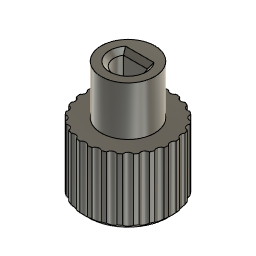
volume-knob (Autodesk Fusion 360 design; units mm, degrees)
Autodesk Fusion 360 part; units mm, degrees
note: some values were not read from the file. Set by a fixed rule: which sketch regions a step uses.
sketch "Skizze1" plane through (0, 0, 0) normal (0, 0, 1) x (1, 0, 0)
  circle A0 centre (0, 0) radius 10
  circle A1 centre (0, 10.5) radius 1
  circle A2 centre (-2.7176, 10.1422) radius 1
  circle A3 centre (-5.25, 9.0933) radius 1
  circle A4 centre (-7.4246, 7.4246) radius 1
  circle A5 centre (-9.0933, 5.25) radius 1
  circle A6 centre (-10.1422, 2.7176) radius 1
  circle A7 centre (-10.5, 0) radius 1
  circle A8 centre (-10.1422, -2.7176) radius 1
  circle A9 centre (-9.0933, -5.25) radius 1
  circle A10 centre (-7.4246, -7.4246) radius 1
  circle A11 centre (-5.25, -9.0933) radius 1
  circle A12 centre (-2.7176, -10.1422) radius 1
  circle A13 centre (0, -10.5) radius 1
  circle A14 centre (2.7176, -10.1422) radius 1
  circle A15 centre (5.25, -9.0933) radius 1
  circle A16 centre (7.4246, -7.4246) radius 1
  circle A17 centre (9.0933, -5.25) radius 1
  circle A18 centre (10.1422, -2.7176) radius 1
  circle A19 centre (10.5, 0) radius 1
  circle A20 centre (10.1422, 2.7176) radius 1
  circle A21 centre (9.0933, 5.25) radius 1
  circle A22 centre (7.4246, 7.4246) radius 1
  circle A23 centre (5.25, 9.0933) radius 1
  circle A24 centre (2.7176, 10.1422) radius 1
  dimension "d1" = 20
  dimension "d2" = 2
  dimension "d4" = 360
  dimension "d7" = 10.5
  constraint coincident A0.centre origin
  measures "d1" diameter of A0
  measures "d2" diameter of A1
  measures "d7" distance of A0.centre A1.centre
extrude "Extrusion1" add sketch "Skizze1" along normal blind 15 contours A0 A1 A2 A3 A4 A5 A6 A7 A8 A9 A10 A11 A12 A13 A14 A15 A16 A17 A18 A19 A20 A21 A22 A23 A24
sketch "Skizze3" plane through (0, 0, 0) normal (0, 1, 0) x (1, 0, 0)
  line L0 (10.9643, -2.0711) -> (7.9643, 0.9289)
  line L1 (7.9643, 0.9289) -> (10.9643, 0.9289)
  line L2 (10.9643, 0.9289) -> (10.9643, -2.0711)
  point P0 (9.9643, 0)
  dimension "d10" = 3
  dimension "d11" = 3
  dimension "d12" = 1
  constraint horizontal L1
  constraint perpendicular L1 L2
  measures "d10" distance of L0.end L1.end
  measures "d11" distance of L0.start L1.end
  measures "d12" distance of L2 P0
revolve "Drehen1" cut sketch "Skizze3" angle 360 about axis through (0, 0, 1.75) along (0, 0, 1)
sketch "Skizze4" plane through (0, 0, 15) normal (0, 0, 1) x (-1, 0, 0)
  arc A0 (-6.4487, -7.6429) -> (-5.7134, -8.2071) centre (0, 0) ccw
  arc A1 (-4.2509, -9.0515) -> (-5.7134, -8.2071) centre (-5.25, -9.0933) ccw
  arc A2 (-4.2509, -9.0515) -> (-3.3946, -9.4062) centre (0, 0) ccw
  arc A3 (-1.7633, -9.8433) -> (-3.3946, -9.4062) centre (-2.7176, -10.1422) ccw
  arc A4 (-1.7633, -9.8433) -> (-0.8444, -9.9643) centre (0, 0) ccw
  arc A5 (0.8444, -9.9643) -> (-0.8444, -9.9643) centre (0, -10.5) ccw
  arc A6 (0.8444, -9.9643) -> (1.7633, -9.8433) centre (0, 0) ccw
  arc A7 (3.3946, -9.4062) -> (1.7633, -9.8433) centre (2.7176, -10.1422) ccw
  arc A8 (3.3946, -9.4062) -> (4.2509, -9.0515) centre (0, 0) ccw
  arc A9 (5.7134, -8.2071) -> (4.2509, -9.0515) centre (5.25, -9.0933) ccw
  arc A10 (5.7134, -8.2071) -> (6.4487, -7.6429) centre (0, 0) ccw
  arc A11 (7.6429, -6.4487) -> (6.4487, -7.6429) centre (7.4246, -7.4246) ccw
  arc A12 (7.6429, -6.4487) -> (8.2071, -5.7134) centre (0, 0) ccw
  arc A13 (9.0515, -4.2509) -> (8.2071, -5.7134) centre (9.0933, -5.25) ccw
  arc A14 (9.0515, -4.2509) -> (9.4062, -3.3946) centre (0, 0) ccw
  arc A15 (9.8433, -1.7633) -> (9.4062, -3.3946) centre (10.1422, -2.7176) ccw
  arc A16 (9.8433, -1.7633) -> (9.9643, -0.8444) centre (0, 0) ccw
  arc A17 (9.9643, 0.8444) -> (9.9643, -0.8444) centre (10.5, 0) ccw
  arc A18 (9.9643, 0.8444) -> (9.8433, 1.7633) centre (0, 0) ccw
  arc A19 (9.4062, 3.3946) -> (9.8433, 1.7633) centre (10.1422, 2.7176) ccw
  arc A20 (9.4062, 3.3946) -> (9.0515, 4.2509) centre (0, 0) ccw
  arc A21 (8.2071, 5.7134) -> (9.0515, 4.2509) centre (9.0933, 5.25) ccw
  arc A22 (8.2071, 5.7134) -> (7.6429, 6.4487) centre (0, 0) ccw
  arc A23 (6.4487, 7.6429) -> (7.6429, 6.4487) centre (7.4246, 7.4246) ccw
  arc A24 (6.4487, 7.6429) -> (5.7134, 8.2071) centre (0, 0) ccw
  arc A25 (4.2509, 9.0515) -> (5.7134, 8.2071) centre (5.25, 9.0933) ccw
  arc A26 (4.2509, 9.0515) -> (3.3946, 9.4062) centre (0, 0) ccw
  arc A27 (1.7633, 9.8433) -> (3.3946, 9.4062) centre (2.7176, 10.1422) ccw
  arc A28 (1.7633, 9.8433) -> (0.8444, 9.9643) centre (0, 0) ccw
  arc A29 (-0.8444, 9.9643) -> (0.8444, 9.9643) centre (0, 10.5) ccw
  arc A30 (-0.8444, 9.9643) -> (-1.7633, 9.8433) centre (0, 0) ccw
  arc A31 (-3.3946, 9.4062) -> (-1.7633, 9.8433) centre (-2.7176, 10.1422) ccw
  arc A32 (-3.3946, 9.4062) -> (-4.2509, 9.0515) centre (0, 0) ccw
  arc A33 (-5.7134, 8.2071) -> (-4.2509, 9.0515) centre (-5.25, 9.0933) ccw
  arc A34 (-5.7134, 8.2071) -> (-6.4487, 7.6429) centre (0, 0) ccw
  arc A35 (-7.6429, 6.4487) -> (-6.4487, 7.6429) centre (-7.4246, 7.4246) ccw
  arc A36 (-7.6429, 6.4487) -> (-8.2071, 5.7134) centre (0, 0) ccw
  arc A37 (-9.0515, 4.2509) -> (-8.2071, 5.7134) centre (-9.0933, 5.25) ccw
  arc A38 (-9.0515, 4.2509) -> (-9.4062, 3.3946) centre (0, 0) ccw
  arc A39 (-9.8433, 1.7633) -> (-9.4062, 3.3946) centre (-10.1422, 2.7176) ccw
  arc A40 (-9.8433, 1.7633) -> (-9.9643, 0.8444) centre (0, 0) ccw
  arc A41 (-9.9643, -0.8444) -> (-9.9643, 0.8444) centre (-10.5, 0) ccw
  arc A42 (-9.9643, -0.8444) -> (-9.8433, -1.7633) centre (0, 0) ccw
  arc A43 (-9.4062, -3.3946) -> (-9.8433, -1.7633) centre (-10.1422, -2.7176) ccw
  arc A44 (-9.4062, -3.3946) -> (-9.0515, -4.2509) centre (0, 0) ccw
  arc A45 (-8.2071, -5.7134) -> (-9.0515, -4.2509) centre (-9.0933, -5.25) ccw
  arc A46 (-8.2071, -5.7134) -> (-7.6429, -6.4487) centre (0, 0) ccw
  arc A47 (-6.4487, -7.6429) -> (-7.6429, -6.4487) centre (-7.4246, -7.4246) ccw
  circle A48 centre (0, 0) radius 6
  dimension "d14" = 12
  constraint concentric A0 A48
  measures "d14" diameter of A48
extrude "Extrusion2" add sketch "Skizze4" along normal blind 11 contours A48
sketch "Skizze5" plane through (0, 0, 26) normal (0, 0, 1) x (-1, 0, 0)
  circle A0 centre (0, 0) radius 6
  circle A1 centre (0, 0) radius 3.15
  line L0 (4, -1.65) -> (-4, -1.65)
  line L1 (0, 3.15) -> (-3, 3.15) construction
  line L2 (0, 3.15) -> (3, 3.15) construction
  dimension "d17" = 6.3
  dimension "d18" = 4.8
  constraint concentric A0 A1
  constraint horizontal L0
  constraint coincident A1 L1.start
  constraint tangent A1 L1
  constraint horizontal L1
  constraint tangent A1 L2
  measures "d17" diameter of A1
  measures "d18" distance of L0 L1
extrude "Extrusion3" cut sketch "Skizze5" against normal blind 24 contours A1 L0 picked at (0.872, -0.5151)
chamfer "Fase1" distance 1 angle 45 2 edges at (0, -3.15, 26) (0, 1.65, 26)
equation "d11 = d10"
